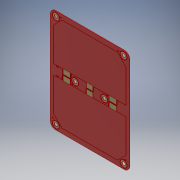
# Autodesk Inventor part: SolarPanel_PCB
Saved by Autodesk Inventor 2018 (Build 220112000, 112)
## iProperties
Created: 2018-05-13
Part Number: SolarPanel_PCB
Material: Fiberglass Batt
Document SubType Name: Modeling
Designer: Bradley
Density: 0.032 g/cm^3
Appearance: Smooth - Red
Author: Bradley
Autodesk Inventor part; units mm, degrees
ref_plane "YZ Plane" through (0, 0, 0) normal (1, 0, 0) x (0, 1, 0)
ref_plane "XZ Plane" through (0, 0, 0) normal (0, 1, 0) x (-1, 0, 0)
ref_plane "XY Plane" through (0, 0, 0) normal (0, 0, 1) x (1, 0, 0)
sketch "Sketch1" plane through (0, 0, 0) normal (0, 1, 0) x (-1, 0, 0)
  line L0 (50, 57) -> (41.5, 57) construction
  line L1 (41.5, 57) -> (41.5, -56.5) construction
  line L2 (41.5, -56.5) -> (50, -56.5) construction
  line L3 (50, -56.5) -> (50, 57) construction
  line L4 (-41.5, 57) -> (-50, 57) construction
  line L5 (-50, 57) -> (-50, -56.5) construction
  line L6 (-50, -56.5) -> (-41.5, -56.5) construction
  line L7 (-41.5, -56.5) -> (-41.5, 57) construction
  line L8 (41.5, 50) -> (-41.5, 50) construction
  line L9 (-41.5, 50) -> (-41.5, -50) construction
  line L10 (-41.5, -50) -> (41.5, -50) construction
  line L11 (41.5, -50) -> (41.5, 50) construction
  line L12 (0, 50) -> (0, -50) construction
  line L13 (33, 49.5) -> (-33, 49.5)
  line L14 (-38, 44.5) -> (-38, -44.5)
  line L15 (-33, -49.5) -> (33, -49.5)
  line L16 (38, -44.5) -> (38, 44.5)
  line L17 (34.5, 5) -> (-34.5, 5) construction
  line L18 (-34.5, 5) -> (-34.5, 36.7) construction
  line L19 (-34.5, 36.7) -> (-26.5, 44.7) construction
  line L20 (-26.5, 44.7) -> (26.5, 44.7) construction
  line L21 (26.5, 44.7) -> (34.5, 36.7) construction
  line L22 (34.5, 36.7) -> (34.5, 5) construction
  line L23 (34.5, -5) -> (-34.5, -5) construction
  line L24 (-34.5, -5) -> (-34.5, -36.7) construction
  line L25 (-34.5, -36.7) -> (-26.5, -44.7) construction
  line L26 (-26.5, -44.7) -> (26.5, -44.7) construction
  line L27 (26.5, -44.7) -> (34.5, -36.7) construction
  line L28 (34.5, -36.7) -> (34.5, -5) construction
  line L29 (0, 5) -> (0, -5) construction
  circle A0 centre (32.5, 45) radius 2.85 construction
  circle A1 centre (32.5, 45) radius 1.65
  circle A2 centre (32.5, 45) radius 1.5 construction
  line L30 (32.5, 45) -> (-32.5, 45) construction
  line L31 (-32.5, 45) -> (-32.5, -45) construction
  line L32 (-32.5, -45) -> (32.5, -45) construction
  line L33 (32.5, -45) -> (32.5, 45) construction
  circle A3 centre (-32.5, -45) radius 1.65
  circle A4 centre (32.5, -45) radius 1.65
  circle A5 centre (-32.5, 45) radius 1.65
  line L34 (14, 0) -> (-14, 0) construction
  circle A6 centre (14, 0) radius 1.65
  circle A7 centre (-14, 0) radius 1.65
  arc A8 (38, 44.5) -> (33, 49.5) centre (33, 44.5) ccw
  arc A9 (-33, 49.5) -> (-38, 44.5) centre (-33, 44.5) ccw
  arc A10 (-38, -44.5) -> (-33, -49.5) centre (-33, -44.5) ccw
  arc A11 (33, -49.5) -> (38, -44.5) centre (33, -44.5) ccw
  point P0 (0, 0)
  point P1 (0, 0)
  point P2 (38, 49.5)
  point P3 (-38, -49.5)
  point P4 (-38, 49.5)
  point P5 (38, -49.5)
  point P6 (0, 49.5)
  point P7 (0, 44.7)
  point P8 (38, 0)
  point P9 (0, 45)
  point P10 (32.5, 0)
  dimension "d0" = 100
  dimension "d1" = 8.5
  dimension "d2" = 100
  dimension "d3" = 6.5
  dimension "d4" = 7
  dimension "d5" = 12
  dimension "d6" = 10
  dimension "d7" = 69
  dimension "d8" = 39.7
  dimension "d10" = 8
  dimension "d11" = 3
  dimension "d12" = 3.3
  dimension "d13" = 5.7
  dimension "d14" = 28
  dimension "d17" = 99
  dimension "d18" = 76
  dimension "d19" = 65
  dimension "d20" = 90
  dimension "d21" = 1.6048
  dimension "d22" = 5
  constraints: 70 end point, 16 point on line, 15 parallel, 12 centre point, 12 midpoint, 9 perpendicular, 8 coincident, 8 equal radius, 8 point on circle, 8 tangent, 7 horizontal, 6 equal length, 3 vertical alignment, 2 horizontal alignment
  measures "d0" distance between parallel lines of L5 L3
  measures "d1" distance of L0.start L0.end
  measures "d2" distance between parallel lines of L10 L8
  measures "d3" distance between parallel lines of L2 L10
  measures "d4" distance between parallel lines of L8 L0
  measures "d5" distance between parallel lines of L16 L3
  measures "d6" distance between parallel lines of L23 L17
  measures "d7" distance of L17.start L17.end
  measures "d8" distance between parallel lines of L17 L20
  measures "d10" horizontal distance of L18.end L19.end
  measures "d11" diameter of A2
  measures "d12" diameter of A1
  measures "d13" diameter of A0
  measures "d14" distance of L34.start L34.end
  measures "d17" distance of point (38, -49.5) point (38, 49.5)
  measures "d18" distance of point (38, 49.5) point (-38, 49.5)
  measures "d19" distance of L30.start L30.end
  measures "d20" distance of L32.end L30.start
  measures "d21" distance edge to line of A0 L21
  measures "d22" radius of A8
extrude "Extrusion1" add sketch "Sketch1" along normal mid plane 0.5
sketch "Sketch2" plane through (0, -0.25, 0) normal (0, -1, 0) x (1, 0, 0)
  line L0 (-18.675, 5) -> (-25.675, 5)
  line L1 (-25.675, 5) -> (-25.675, 0.5)
  line L2 (-25.675, 0.5) -> (-18.675, 0.5)
  line L3 (-18.675, 0.5) -> (-18.675, 5)
  line L4 (3, 5) -> (-3, 5)
  line L5 (-3, 5) -> (-3, 0.5)
  line L6 (-3, 0.5) -> (3, 0.5)
  line L7 (3, 0.5) -> (3, 5)
  line L8 (18.675, 5) -> (25.675, 5)
  line L9 (25.675, 5) -> (25.675, 0.5)
  line L10 (25.675, 0.5) -> (18.675, 0.5)
  line L11 (18.675, 0.5) -> (18.675, 5)
  line L12 (-22.175, 5) -> (22.175, 5) construction
  line L13 (-25.675, 0) -> (25.675, 0)
  line L14 (-18.675, -5) -> (-25.675, -5)
  line L15 (-25.675, -5) -> (-25.675, -0.5)
  line L16 (-25.675, -0.5) -> (-18.675, -0.5)
  line L17 (-18.675, -0.5) -> (-18.675, -5)
  line L18 (3, -5) -> (-3, -5)
  line L19 (-3, -5) -> (-3, -0.5)
  line L20 (-3, -0.5) -> (3, -0.5)
  line L21 (3, -0.5) -> (3, -5)
  line L22 (18.675, -5) -> (25.675, -5)
  line L23 (25.675, -5) -> (25.675, -0.5)
  line L24 (25.675, -0.5) -> (18.675, -0.5)
  line L25 (18.675, -0.5) -> (18.675, -5)
  circle A0 centre (14, 0) radius 1.65 projected
  circle A1 centre (-14, 0) radius 1.65 projected
  circle A2 centre (32.5, 45) radius 1.65 projected
  circle A3 centre (-32.5, -45) radius 1.65 projected
  circle A4 centre (32.5, -45) radius 1.65 projected
  circle A5 centre (-32.5, 45) radius 1.65 projected
  line L26 (33, 49.5) -> (-33, 49.5) projected
  arc A6 (-33, 49.5) -> (-38, 44.5) centre (-33, 44.5) ccw projected
  line L27 (-38, 44.5) -> (-38, -44.5) projected
  arc A7 (-38, -44.5) -> (-33, -49.5) centre (-33, -44.5) ccw projected
  line L28 (-33, -49.5) -> (33, -49.5) projected
  arc A8 (33, -49.5) -> (38, -44.5) centre (33, -44.5) ccw projected
  line L29 (38, -44.5) -> (38, 44.5) projected
  arc A9 (38, 44.5) -> (33, 49.5) centre (33, 44.5) ccw projected
  circle A10 centre (-14, 0) radius 3
  circle A11 centre (14, 0) radius 3
  circle A12 centre (-32.5, 45) radius 3
  circle A13 centre (32.5, 45) radius 1.65 projected
  circle A14 centre (32.5, 45) radius 3
  circle A15 centre (-32.5, -45) radius 1.65 projected
  circle A16 centre (-32.5, -45) radius 3
  circle A17 centre (32.5, -45) radius 1.65 projected
  circle A18 centre (32.5, -45) radius 3
  point P0 (0, 0)
  point P1 (0, 5)
  point P2 (0, 0)
  dimension "d23" = 44.35
  dimension "d24" = 7
  dimension "d25" = 4.5
  dimension "d26" = 6
  dimension "d27" = 5
  dimension "d47" = 6
  constraints: 52 end point, 12 symmetric about line, 9 point on line, 7 coincident, 7 parallel, 6 centre point, 5 equal radius, 5 midpoint, 3 horizontal, 3 perpendicular, 2 collinear, 1 horizontal alignment, 1 vertical alignment
  measures "d23" distance of L12.end L12.start
  measures "d24" distance of L1.end L2.end
  measures "d25" distance of L0.end L1.end
  measures "d26" distance of L5.end L6.end
  measures "d27" distance from line of point (0, 0) L12
  measures "d47" diameter of A10
extrude "Extrusion2" add sketch "Sketch2" along normal blind 0.035 contours L3 L2 L1 L0 | L7 L6 L5 L4 | L8 L9 L10 L11 | A1 L13 A10 | L13 A10 A1 | A0 L13 A11 | L13 A11 A0 | L14 L15 L16 L17 | L18 L19 L20 L21 | L25 L24 L23 L22 | A12 | A14 | A16 | A18
sketch "Sketch3" plane through (0, -0.25, 0) normal (0, -1, 0) x (1, 0, 0)
  line L0 (-25.675, -5) -> (-25.675, -0.5) projected
  line L1 (-25.675, -0.5) -> (-18.675, -0.5) projected
  line L2 (-18.675, -0.5) -> (-18.675, -5) projected
  line L3 (-18.675, -5) -> (-25.675, -5) projected
  line L4 (-18.675, 5) -> (-18.675, 0.5) projected
  line L5 (-18.675, 0.5) -> (-25.675, 0.5) projected
  line L6 (-25.675, 0.5) -> (-25.675, 5) projected
  line L7 (-25.675, 5) -> (-18.675, 5) projected
  line L8 (3, 5) -> (3, 0.5) projected
  line L9 (3, 0.5) -> (-3, 0.5) projected
  line L10 (-3, 0.5) -> (-3, 5) projected
  line L11 (-3, 5) -> (3, 5) projected
  line L12 (-3, -5) -> (-3, -0.5) projected
  line L13 (-3, -0.5) -> (3, -0.5) projected
  line L14 (3, -0.5) -> (3, -5) projected
  line L15 (3, -5) -> (-3, -5) projected
  line L16 (25.675, 5) -> (25.675, 0.5) projected
  line L17 (25.675, 0.5) -> (18.675, 0.5) projected
  line L18 (18.675, 0.5) -> (18.675, 5) projected
  line L19 (18.675, 5) -> (25.675, 5) projected
  line L20 (25.675, -0.5) -> (25.675, -5) projected
  line L21 (25.675, -5) -> (18.675, -5) projected
  line L22 (18.675, -5) -> (18.675, -0.5) projected
  line L23 (18.675, -0.5) -> (25.675, -0.5) projected
  line L24 (33, 49.5) -> (-33, 49.5) projected
  arc A0 (-33, 49.5) -> (-38, 44.5) centre (-33, 44.5) ccw projected
  line L25 (-38, 44.5) -> (-38, -44.5) projected
  arc A1 (-38, -44.5) -> (-33, -49.5) centre (-33, -44.5) ccw projected
  line L26 (-33, -49.5) -> (33, -49.5) projected
  arc A2 (33, -49.5) -> (38, -44.5) centre (33, -44.5) ccw projected
  line L27 (38, -44.5) -> (38, 44.5) projected
  arc A3 (38, 44.5) -> (33, 49.5) centre (33, 44.5) ccw projected
  circle A4 centre (-18.1, 3.824) radius 0.225
  circle A5 centre (-18.1, 1.676) radius 0.225
  circle A6 centre (-18.1, 2.75) radius 0.225
  line L28 (-18.675, 5) -> (-17.7995, 4.1245)
  arc A7 (-17.675, 3.824) -> (-17.7995, 4.1245) centre (-18.1, 3.824) ccw
  line L29 (-17.675, 3.824) -> (-17.675, 1.676)
  arc A8 (-17.7995, 1.3755) -> (-17.675, 1.676) centre (-18.1, 1.676) ccw
  line L30 (-17.7995, 1.3755) -> (-18.675, 0.5)
  line L31 (-18.1, 3.824) -> (-18.1, 1.676) construction
  line L32 (-18.675, 5) -> (-18.675, 0.5)
  line L33 (3, 5) -> (3, 0.5) construction
  line L34 (3, 5) -> (3.8755, 4.1245)
  arc A9 (4, 3.824) -> (3.8755, 4.1245) centre (3.575, 3.824) ccw
  line L35 (4, 3.824) -> (4, 1.676)
  arc A10 (3.8755, 1.3755) -> (4, 1.676) centre (3.575, 1.676) ccw
  line L36 (3.8755, 1.3755) -> (3, 0.5)
  line L37 (25.675, 0.5) -> (26.5505, 1.3755)
  arc A11 (26.5505, 1.3755) -> (26.675, 1.676) centre (26.25, 1.676) ccw
  line L38 (26.675, 1.676) -> (26.675, 3.824)
  arc A12 (26.675, 3.824) -> (26.5505, 4.1245) centre (26.25, 3.824) ccw
  line L39 (26.5505, 4.1245) -> (25.675, 5)
  line L40 (3, 5) -> (3, 0.5)
  line L41 (25.675, 5) -> (25.675, 0.5)
  line L42 (-4, -3.824) -> (-4, -1.676)
  arc A13 (-4, -3.824) -> (-3.8755, -4.1245) centre (-3.575, -3.824) ccw
  arc A14 (-3.8755, -1.3755) -> (-4, -1.676) centre (-3.575, -1.676) ccw
  line L43 (-25.675, -5) -> (-25.675, -0.5)
  line L44 (-25.675, -0.5) -> (-26.5505, -1.3755)
  arc A15 (-26.675, -3.824) -> (-26.5505, -4.1245) centre (-26.25, -3.824) ccw
  line L45 (-26.675, -1.676) -> (-26.675, -3.824)
  arc A16 (-26.5505, -1.3755) -> (-26.675, -1.676) centre (-26.25, -1.676) ccw
  line L46 (-26.5505, -4.1245) -> (-25.675, -5)
  circle A17 centre (18.1, -3.824) radius 0.225
  circle A18 centre (18.1, -1.676) radius 0.225
  circle A19 centre (18.1, -2.75) radius 0.225
  line L47 (18.675, -5) -> (17.7995, -4.1245)
  arc A20 (17.675, -3.824) -> (17.7995, -4.1245) centre (18.1, -3.824) ccw
  line L48 (-3, -5) -> (-3.8755, -4.1245)
  line L49 (-3.8755, -1.3755) -> (-3, -0.5)
  line L50 (17.675, -3.824) -> (17.675, -1.676)
  arc A21 (17.7995, -1.3755) -> (17.675, -1.676) centre (18.1, -1.676) ccw
  line L51 (18.1, -3.824) -> (18.1, -1.676) construction
  line L52 (17.7995, -1.3755) -> (18.675, -0.5)
  line L53 (18.675, -5) -> (18.675, -0.5)
  line L54 (-3, -5) -> (-3, -0.5)
  line L55 (3.575, 3.824) -> (3.575, 1.676) construction
  line L56 (26.25, 3.824) -> (26.25, 1.676) construction
  line L57 (-3.575, -1.676) -> (-3.575, -3.824) construction
  line L58 (-26.25, -1.676) -> (-26.25, -3.824) construction
  circle A22 centre (3.575, 3.824) radius 0.225
  circle A23 centre (3.575, 2.75) radius 0.225
  circle A24 centre (3.575, 1.676) radius 0.225
  circle A25 centre (26.25, 3.824) radius 0.225
  circle A26 centre (26.25, 2.75) radius 0.225
  circle A27 centre (26.25, 1.676) radius 0.225
  circle A28 centre (-3.575, -1.676) radius 0.225
  circle A29 centre (-3.575, -2.75) radius 0.225
  circle A30 centre (-3.575, -3.824) radius 0.225
  circle A31 centre (-26.25, -1.676) radius 0.225
  circle A32 centre (-26.25, -2.75) radius 0.225
  circle A33 centre (-26.25, -3.824) radius 0.225
  circle A34 centre (-14, 0) radius 3 projected
  circle A35 centre (-14, 0) radius 3.5 construction
  point P0 (0, 0)
  dimension "d30" = 0.45
  dimension "d31" = 45
  dimension "d32" = 0.2
  dimension "d33" = 1
  dimension "d36" = 360
  dimension "d48" = 7
  constraints: 60 end point, 31 centre point, 24 point on circle, 19 equal radius, 15 coincident, 12 tangent, 7 equal length, 7 vertical, 5 midpoint, 2 collinear, 2 parallel, 101 other
  measures "d30" diameter of A4
  measures "d31" angle of L4 L28
  measures "d32" radial gap between concentric circles of A4 A7
  measures "d33" distance between parallel lines of L4 L29
  measures "d48" diameter of A35
extrude "Extrusion3" add sketch "Sketch3" along normal blind 0.05 contours L46 A15 L45 A16 L44 L0 | L28 A7 L29 A8 L30 L4 | L34 A9 L35 A10 L36 L8 | L48 A13 L42 A14 L49 L12 | L39 A12 L38 A11 L37 L16 | L22 L47 A20 L50 A21 L52
sketch "Sketch6" plane through (0, -0.25, 0) normal (0, -1, 0) x (1, 0, 0)
  line L0 (33, 49.5) -> (-33, 49.5) projected
  arc A0 (-33, 49.5) -> (-38, 44.5) centre (-33, 44.5) ccw projected
  line L1 (-38, 44.5) -> (-38, -44.5) projected
  arc A1 (-38, -44.5) -> (-33, -49.5) centre (-33, -44.5) ccw projected
  line L2 (-33, -49.5) -> (33, -49.5) projected
  arc A2 (33, -49.5) -> (38, -44.5) centre (33, -44.5) ccw projected
  line L3 (38, -44.5) -> (38, 44.5) projected
  arc A3 (38, 44.5) -> (33, 49.5) centre (33, 44.5) ccw projected
  line L4 (25.675, 5) -> (26.5505, 4.1245) projected
  arc A4 (26.675, 3.824) -> (26.5505, 4.1245) centre (26.25, 3.824) ccw projected
  line L5 (26.675, 3.824) -> (26.675, 1.676) projected
  arc A5 (26.5505, 1.3755) -> (26.675, 1.676) centre (26.25, 1.676) ccw projected
  line L6 (26.5505, 1.3755) -> (25.675, 0.5) projected
  line L7 (25.675, 0.5) -> (18.675, 0.5) projected
  line L8 (18.675, 0.5) -> (18.675, 5) projected
  line L9 (18.675, 5) -> (25.675, 5) projected
  circle A6 centre (32.5, -45) radius 3 projected
  circle A7 centre (32.5, 45) radius 3 projected
  circle A8 centre (14, 0) radius 3 projected
  line L10 (3, 5) -> (3.8755, 4.1245) projected
  arc A9 (4, 3.824) -> (3.8755, 4.1245) centre (3.575, 3.824) ccw projected
  line L11 (4, 3.824) -> (4, 1.676) projected
  arc A10 (3.8755, 1.3755) -> (4, 1.676) centre (3.575, 1.676) ccw projected
  line L12 (3.8755, 1.3755) -> (3, 0.5) projected
  line L13 (3, 0.5) -> (-3, 0.5) projected
  line L14 (-3, 0.5) -> (-3, 5) projected
  line L15 (-3, 5) -> (3, 5) projected
  circle A11 centre (-14, 0) radius 3 projected
  circle A12 centre (-32.5, 45) radius 3 projected
  circle A13 centre (-32.5, -45) radius 3 projected
  line L16 (-18.675, 5) -> (-17.7995, 4.1245) projected
  arc A14 (-17.675, 3.824) -> (-17.7995, 4.1245) centre (-18.1, 3.824) ccw projected
  line L17 (-17.675, 3.824) -> (-17.675, 1.676) projected
  arc A15 (-17.7995, 1.3755) -> (-17.675, 1.676) centre (-18.1, 1.676) ccw projected
  line L18 (-17.7995, 1.3755) -> (-18.675, 0.5) projected
  line L19 (-18.675, 0.5) -> (-25.675, 0.5) projected
  line L20 (-25.675, 0.5) -> (-25.675, 5) projected
  line L21 (-25.675, 5) -> (-18.675, 5) projected
  line L22 (17.7995, -1.3755) -> (18.675, -0.5) projected
  line L23 (18.675, -0.5) -> (25.675, -0.5) projected
  line L24 (25.675, -0.5) -> (25.675, -5) projected
  line L25 (25.675, -5) -> (18.675, -5) projected
  line L26 (18.675, -5) -> (17.7995, -4.1245) projected
  arc A16 (17.675, -3.824) -> (17.7995, -4.1245) centre (18.1, -3.824) ccw projected
  line L27 (17.675, -3.824) -> (17.675, -1.676) projected
  arc A17 (17.7995, -1.3755) -> (17.675, -1.676) centre (18.1, -1.676) ccw projected
  line L28 (-3.8755, -1.3755) -> (-3, -0.5) projected
  line L29 (-3, -0.5) -> (3, -0.5) projected
  line L30 (3, -0.5) -> (3, -5) projected
  line L31 (3, -5) -> (-3, -5) projected
  line L32 (-3, -5) -> (-3.8755, -4.1245) projected
  arc A18 (-4, -3.824) -> (-3.8755, -4.1245) centre (-3.575, -3.824) ccw projected
  line L33 (-4, -3.824) -> (-4, -1.676) projected
  arc A19 (-3.8755, -1.3755) -> (-4, -1.676) centre (-3.575, -1.676) ccw projected
  line L34 (-26.5505, -1.3755) -> (-25.675, -0.5) projected
  line L35 (-25.675, -0.5) -> (-18.675, -0.5) projected
  line L36 (-18.675, -0.5) -> (-18.675, -5) projected
  line L37 (-18.675, -5) -> (-25.675, -5) projected
  line L38 (-25.675, -5) -> (-26.5505, -4.1245) projected
  arc A20 (-26.675, -3.824) -> (-26.5505, -4.1245) centre (-26.25, -3.824) ccw projected
  line L39 (-26.675, -3.824) -> (-26.675, -1.676) projected
  arc A21 (-26.5505, -1.3755) -> (-26.675, -1.676) centre (-26.25, -1.676) ccw projected
  circle A22 centre (-14, 0) radius 3.5 construction
  circle A23 centre (14, 0) radius 3.5 construction
  circle A24 centre (32.5, 45) radius 1.65 construction
  circle A25 centre (32.5, 45) radius 3.5 construction
  circle A26 centre (-32.5, 45) radius 3.5 construction
  circle A27 centre (-32.5, -45) radius 1.65 construction
  circle A28 centre (-32.5, -45) radius 3.5 construction
  circle A29 centre (32.5, -45) radius 1.65 construction
  circle A30 centre (32.5, -45) radius 3.5 construction
  line L40 (-34.75, 4.75) -> (-25.925, 4.75) construction
  line L41 (-25.925, 4.75) -> (-25.925, 0.25) construction
  line L42 (-25.925, 0.25) -> (-18.425, 0.25) construction
  line L43 (-18.425, 0.25) -> (-18.425, 4.75) construction
  line L44 (-18.425, 4.75) -> (-3.25, 4.75) construction
  line L45 (-3.25, 4.75) -> (-3.25, 0.25) construction
  line L46 (-3.25, 0.25) -> (3.25, 0.25) construction
  line L47 (3.25, 0.25) -> (3.25, 4.75) construction
  line L48 (3.25, 4.75) -> (18.425, 4.75) construction
  line L49 (18.425, 4.75) -> (18.425, 0.25) construction
  line L50 (18.425, 0.25) -> (25.925, 0.25) construction
  line L51 (25.925, 0.25) -> (25.925, 4.75) construction
  line L52 (25.925, 4.75) -> (34.75, 4.75) construction
  line L53 (34.75, 4.75) -> (34.75, 36.8036) construction
  line L54 (34.75, 36.8036) -> (26.6036, 44.95) construction
  line L55 (26.6036, 44.95) -> (-26.6036, 44.95) construction
  line L56 (-26.6036, 44.95) -> (-34.75, 36.8036) construction
  line L57 (-34.75, 36.8036) -> (-34.75, 4.75) construction
  line L58 (-25.675, 0.5) -> (-18.675, 0.5) construction
  line L59 (-3, 0.5) -> (3, 0.5) construction
  line L60 (18.675, 0.5) -> (25.675, 0.5) construction
  line L61 (-34.5, 36.7) -> (-34.5, 5) construction
  line L62 (-26.5, 44.7) -> (-34.5, 36.7) construction
  line L63 (26.5, 44.7) -> (-26.5, 44.7) construction
  line L64 (34.5, 36.7) -> (26.5, 44.7) construction
  line L65 (34.5, 5) -> (34.5, 36.7) construction
  line L66 (-26.6346, 45.025) -> (26.6346, 45.025)
  line L67 (26.6346, 45.025) -> (34.825, 36.8346)
  line L68 (34.825, 36.8346) -> (34.825, 4.675)
  line L69 (34.825, 4.675) -> (26, 4.675)
  line L70 (26, 4.675) -> (26, 0.175)
  line L71 (26, 0.175) -> (18.35, 0.175)
  line L72 (18.35, 0.175) -> (18.35, 4.675)
  line L73 (18.35, 4.675) -> (3.325, 4.675)
  line L74 (3.325, 4.675) -> (3.325, 0.175)
  line L75 (3.325, 0.175) -> (-3.325, 0.175)
  line L76 (-3.325, 0.175) -> (-3.325, 4.675)
  line L77 (-3.325, 4.675) -> (-18.35, 4.675)
  line L78 (-18.35, 4.675) -> (-18.35, 0.175)
  line L79 (-18.35, 0.175) -> (-26, 0.175)
  line L80 (-26, 0.175) -> (-26, 4.675)
  line L81 (-26, 4.675) -> (-34.825, 4.675)
  line L82 (-34.825, 4.675) -> (-34.825, 36.8346)
  line L83 (-34.825, 36.8346) -> (-26.6346, 45.025)
  line L84 (-26.5725, 44.875) -> (26.5725, 44.875)
  line L85 (26.5725, 44.875) -> (34.675, 36.7725)
  line L86 (34.675, 36.7725) -> (34.675, 4.825)
  line L87 (34.675, 4.825) -> (25.85, 4.825)
  line L88 (25.85, 4.825) -> (25.85, 0.325)
  line L89 (25.85, 0.325) -> (18.5, 0.325)
  line L90 (18.5, 0.325) -> (18.5, 4.825)
  line L91 (18.5, 4.825) -> (3.175, 4.825)
  line L92 (3.175, 4.825) -> (3.175, 0.325)
  line L93 (3.175, 0.325) -> (-3.175, 0.325)
  line L94 (-3.175, 0.325) -> (-3.175, 4.825)
  line L95 (-3.175, 4.825) -> (-18.5, 4.825)
  line L96 (-18.5, 4.825) -> (-18.5, 0.325)
  line L97 (-18.5, 0.325) -> (-25.85, 0.325)
  line L98 (-25.85, 0.325) -> (-25.85, 4.825)
  line L99 (-25.85, 4.825) -> (-34.675, 4.825)
  line L100 (-34.675, 4.825) -> (-34.675, 36.7725)
  line L101 (-34.675, 36.7725) -> (-26.5725, 44.875)
  line L102 (-14, 0) -> (14, 0) construction
  line L103 (-34.675, -4.825) -> (-25.85, -4.825)
  line L104 (-34.825, -4.675) -> (-26, -4.675)
  line L105 (-34.675, -36.7725) -> (-34.675, -4.825)
  line L106 (-34.825, -36.8346) -> (-34.825, -4.675)
  line L107 (-34.75, -4.75) -> (-34.75, -36.8036) construction
  line L108 (-25.925, -4.75) -> (-34.75, -4.75) construction
  line L109 (3.325, -4.675) -> (18.35, -4.675)
  line L110 (18.425, -4.75) -> (3.25, -4.75) construction
  line L111 (3.175, -4.825) -> (18.5, -4.825)
  line L112 (3.25, -4.75) -> (3.25, -0.25) construction
  line L113 (3.25, -0.25) -> (-3.25, -0.25) construction
  line L114 (-3.325, -0.175) -> (3.325, -0.175)
  line L115 (-25.85, -4.825) -> (-25.85, -0.325)
  line L116 (-25.85, -0.325) -> (-18.5, -0.325)
  line L117 (-3.325, -4.675) -> (-3.325, -0.175)
  line L118 (-18.35, -4.675) -> (-3.325, -4.675)
  line L119 (-18.35, -0.175) -> (-18.35, -4.675)
  line L120 (-18.5, -0.325) -> (-18.5, -4.825)
  line L121 (-18.5, -4.825) -> (-3.175, -4.825)
  line L122 (-3.175, -4.825) -> (-3.175, -0.325)
  line L123 (-3.25, -0.25) -> (-3.25, -4.75) construction
  line L124 (-3.25, -4.75) -> (-18.425, -4.75) construction
  line L125 (-18.425, -4.75) -> (-18.425, -0.25) construction
  line L126 (-25.925, -0.25) -> (-25.925, -4.75) construction
  line L127 (-26, -4.675) -> (-26, -0.175)
  line L128 (-18.425, -0.25) -> (-25.925, -0.25) construction
  line L129 (18.425, -0.25) -> (18.425, -4.75) construction
  line L130 (18.35, -4.675) -> (18.35, -0.175)
  line L131 (18.5, -0.325) -> (25.85, -0.325)
  line L132 (25.925, -0.25) -> (18.425, -0.25) construction
  line L133 (18.35, -0.175) -> (26, -0.175)
  line L134 (25.85, -0.325) -> (25.85, -4.825)
  line L135 (25.925, -4.75) -> (25.925, -0.25) construction
  line L136 (26, -0.175) -> (26, -4.675)
  line L137 (26.6346, -45.025) -> (-26.6346, -45.025)
  line L138 (34.675, -4.825) -> (34.675, -36.7725)
  line L139 (34.75, -36.8036) -> (34.75, -4.75) construction
  line L140 (34.825, -4.675) -> (34.825, -36.8346)
  line L141 (18.5, -4.825) -> (18.5, -0.325)
  line L142 (26.5725, -44.875) -> (-26.5725, -44.875)
  line L143 (-26.6036, -44.95) -> (26.6036, -44.95) construction
  line L144 (34.75, -4.75) -> (25.925, -4.75) construction
  line L145 (25.85, -4.825) -> (34.675, -4.825)
  line L146 (26, -4.675) -> (34.825, -4.675)
  line L147 (-26, -0.175) -> (-18.35, -0.175)
  line L148 (34.675, -36.7725) -> (26.5725, -44.875)
  line L149 (26.6036, -44.95) -> (34.75, -36.8036) construction
  line L150 (34.825, -36.8346) -> (26.6346, -45.025)
  line L151 (-26.5725, -44.875) -> (-34.675, -36.7725)
  line L152 (-34.75, -36.8036) -> (-26.6036, -44.95) construction
  line L153 (-26.6346, -45.025) -> (-34.825, -36.8346)
  line L154 (3.175, -0.325) -> (3.175, -4.825)
  line L155 (3.325, -0.175) -> (3.325, -4.675)
  line L156 (-3.175, -0.325) -> (3.175, -0.325)
  circle A31 centre (-14, 0) radius 3.575
  circle A32 centre (-14, 0) radius 3.425
  circle A33 centre (14, 0) radius 3.575
  circle A34 centre (14, 0) radius 3.425
  circle A35 centre (32.5, 45) radius 3.575
  circle A36 centre (32.5, 45) radius 3.425
  circle A37 centre (-32.5, 45) radius 3.575
  circle A38 centre (-32.5, 45) radius 3.425
  circle A39 centre (32.5, -45) radius 3.575
  circle A40 centre (32.5, -45) radius 3.425
  circle A41 centre (-32.5, -45) radius 3.575
  circle A42 centre (-32.5, -45) radius 3.425
  line L157 (-32.0298, 4.2303) -> (-29.8638, 4.2303) construction
  line L158 (-29.8638, 4.2303) -> (-29.8638, 3.4284) construction
  line L159 (-29.8638, 3.4284) -> (-32.0298, 3.4284) construction
  line L160 (-32.0298, 3.4284) -> (-32.0298, 4.2303) construction
  line L161 (-32.0692, -3.4048) -> (-29.9032, -3.4048) construction
  line L162 (-29.9032, -3.4048) -> (-29.9032, -4.2067) construction
  line L163 (-29.9032, -4.2067) -> (-32.0692, -4.2067) construction
  line L164 (-32.0692, -4.2067) -> (-32.0692, -3.4048) construction
  line L165 (-17.5305, -3.2221) -> (-15.3645, -3.2221) construction
  line L166 (-15.3645, -3.2221) -> (-15.3645, -4.024) construction
  line L167 (-15.3645, -4.024) -> (-17.5305, -4.024) construction
  line L168 (-17.5305, -4.024) -> (-17.5305, -3.2221) construction
  line L169 (15.9624, 4.2512) -> (18.1284, 4.2512) construction
  line L170 (18.1284, 4.2512) -> (18.1284, 3.4492) construction
  line L171 (18.1284, 3.4492) -> (15.9624, 3.4492) construction
  line L172 (15.9624, 3.4492) -> (15.9624, 4.2512) construction
  line L173 (-28.7606, 46.6145) -> (-26.5946, 46.6145) construction
  line L174 (-26.5946, 46.6145) -> (-26.5946, 45.8126) construction
  line L175 (-26.5946, 45.8126) -> (-28.7606, 45.8126) construction
  line L176 (-28.7606, 45.8126) -> (-28.7606, 46.6145) construction
  line L177 (26.5067, 46.7387) -> (28.6727, 46.7387) construction
  line L178 (28.6727, 46.7387) -> (28.6727, 45.9367) construction
  line L179 (28.6727, 45.9367) -> (26.5067, 45.9367) construction
  line L180 (26.5067, 45.9367) -> (26.5067, 46.7387) construction
  line L181 (-36.2344, -40.3855) -> (-34.0684, -40.3855) construction
  line L182 (-34.0684, -40.3855) -> (-34.0684, -41.1874) construction
  line L183 (-34.0684, -41.1874) -> (-36.2344, -41.1874) construction
  line L184 (-36.2344, -41.1874) -> (-36.2344, -40.3855) construction
  line L185 (33.6109, -40.4304) -> (35.7769, -40.4304) construction
  line L186 (35.7769, -40.4304) -> (35.7769, -41.2324) construction
  line L187 (35.7769, -41.2324) -> (33.6109, -41.2324) construction
  line L188 (33.6109, -41.2324) -> (33.6109, -40.4304) construction
  line L189 (-28.0027, 45.8126) -> (-28.2037, 45.8126)
  line L190 (-28.2037, 45.8126) -> (-28.2037, 46.1672)
  line L191 (-28.2037, 46.1672) -> (-28.4766, 46.1672)
  line L192 (-28.4766, 46.1672) -> (-28.4766, 45.8126)
  line L193 (-28.4766, 45.8126) -> (-28.6776, 45.8126)
  line L194 (-28.6776, 45.8126) -> (-28.6776, 46.6126)
  line L195 (-28.6776, 46.6126) -> (-28.4766, 46.6126)
  line L196 (-28.4766, 46.6126) -> (-28.4766, 46.3196)
  line L197 (-28.4766, 46.3196) -> (-28.2037, 46.3196)
  line L198 (-28.2037, 46.3196) -> (-28.2037, 46.6126)
  line L199 (-28.2037, 46.6126) -> (-28.0027, 46.6126)
  line L200 (-28.0027, 46.6126) -> (-28.0027, 45.8126)
  line L201 (-27.2863, 45.8126) -> (-27.8147, 45.8126)
  line L202 (-27.8147, 45.8126) -> (-27.8147, 45.952)
  line L203 (-27.8147, 45.952) -> (-27.6461, 45.952)
  line L204 (-27.6461, 45.952) -> (-27.6461, 46.3753)
  line L205 (-27.6461, 46.3753) -> (-27.8147, 46.3753)
  line L206 (-27.8147, 46.3753) -> (-27.8147, 46.5056)
  spline S0 degree 2 poles (-27.8147, 46.5056) (-27.7777, 46.5056) (-27.7045, 46.5154) (-27.6824, 46.5257) knots 0 0 0 1 2 2 2
  spline S1 degree 2 poles (-27.6824, 46.5257) (-27.6571, 46.5387) (-27.6286, 46.5821) (-27.626, 46.6145) knots 0 0 0 1 2 2 2
  line L207 (-27.626, 46.6145) -> (-27.451, 46.6145)
  line L208 (-27.451, 46.6145) -> (-27.451, 45.952)
  line L209 (-27.451, 45.952) -> (-27.2863, 45.952)
  line L210 (-27.2863, 45.952) -> (-27.2863, 45.8126)
  line L211 (27.2646, 45.9231) -> (27.0636, 45.9231)
  line L212 (27.0636, 45.9231) -> (27.0636, 46.2777)
  line L213 (27.0636, 46.2777) -> (26.7907, 46.2777)
  line L214 (26.7907, 46.2777) -> (26.7907, 45.9231)
  line L215 (26.7907, 45.9231) -> (26.5897, 45.9231)
  line L216 (26.5897, 45.9231) -> (26.5897, 46.7231)
  line L217 (26.5897, 46.7231) -> (26.7907, 46.7231)
  line L218 (26.7907, 46.7231) -> (26.7907, 46.4301)
  line L219 (26.7907, 46.4301) -> (27.0636, 46.4301)
  line L220 (27.0636, 46.4301) -> (27.0636, 46.7231)
  line L221 (27.0636, 46.7231) -> (27.2646, 46.7231)
  line L222 (27.2646, 46.7231) -> (27.2646, 45.9231)
  line L223 (28.0166, 45.9231) -> (27.4286, 45.9231)
  line L224 (27.4286, 45.9231) -> (27.4286, 46.0534)
  spline S2 degree 2 poles (27.4286, 46.0534) (27.5032, 46.1131) (27.6224, 46.2181) (27.6672, 46.2654) knots 0 0 0 1 2 2 2
  spline S3 degree 2 poles (27.6672, 46.2654) (27.7262, 46.327) (27.7787, 46.421) (27.7787, 46.4703) knots 0 0 0 1 2 2 2
  spline S4 degree 2 poles (27.7787, 46.4703) (27.7787, 46.526) (27.7119, 46.5857) (27.6523, 46.5857) knots 0 0 0 1 2 2 2
  spline S5 degree 2 poles (27.6523, 46.5857) (27.6218, 46.5857) (27.5673, 46.5708) (27.5395, 46.5591) knots 0 0 0 1 2 2 2
  spline S6 degree 2 poles (27.5395, 46.5591) (27.5122, 46.5468) (27.4733, 46.5209) (27.4636, 46.5144) knots 0 0 0 1 2 2 2
  line L225 (27.4636, 46.5144) -> (27.448, 46.5144)
  line L226 (27.448, 46.5144) -> (27.448, 46.6888)
  spline S7 degree 2 poles (27.448, 46.6888) (27.4818, 46.705) (27.6257, 46.7387) (27.6925, 46.7387) knots 0 0 0 1 2 2 2
  spline S8 degree 2 poles (27.6925, 46.7387) (27.8351, 46.7387) (27.9816, 46.6116) (27.9816, 46.4969) knots 0 0 0 1 2 2 2
  spline S9 degree 2 poles (27.9816, 46.4969) (27.9816, 46.4262) (27.9148, 46.2901) (27.8377, 46.2123) knots 0 0 0 1 2 2 2
  spline S10 degree 2 poles (27.8377, 46.2123) (27.7891, 46.1643) (27.6976, 46.0897) (27.6775, 46.0742) knots 0 0 0 1 2 2 2
  line L227 (27.6775, 46.0742) -> (28.0166, 46.0742)
  line L228 (28.0166, 46.0742) -> (28.0166, 45.9231)
  line L229 (16.7203, 3.4512) -> (16.5193, 3.4512)
  line L230 (16.5193, 3.4512) -> (16.5193, 3.8058)
  line L231 (16.5193, 3.8058) -> (16.2464, 3.8058)
  line L232 (16.2464, 3.8058) -> (16.2464, 3.4512)
  line L233 (16.2464, 3.4512) -> (16.0454, 3.4512)
  line L234 (16.0454, 3.4512) -> (16.0454, 4.2512)
  line L235 (16.0454, 4.2512) -> (16.2464, 4.2512)
  line L236 (16.2464, 4.2512) -> (16.2464, 3.9581)
  line L237 (16.2464, 3.9581) -> (16.5193, 3.9581)
  line L238 (16.5193, 3.9581) -> (16.5193, 4.2512)
  line L239 (16.5193, 4.2512) -> (16.7203, 4.2512)
  line L240 (16.7203, 4.2512) -> (16.7203, 3.4512)
  line L241 (17.482, 3.6379) -> (17.3738, 3.6379)
  line L242 (17.3738, 3.6379) -> (17.3738, 3.4492)
  line L243 (17.3738, 3.4492) -> (17.1799, 3.4492)
  line L244 (17.1799, 3.4492) -> (17.1799, 3.6379)
  line L245 (17.1799, 3.6379) -> (16.8273, 3.6379)
  line L246 (16.8273, 3.6379) -> (16.8273, 3.787)
  line L247 (16.8273, 3.787) -> (17.1734, 4.2512)
  line L248 (17.1734, 4.2512) -> (17.3738, 4.2512)
  line L249 (17.3738, 4.2512) -> (17.3738, 3.7818)
  line L250 (17.3738, 3.7818) -> (17.482, 3.7818)
  line L251 (17.482, 3.7818) -> (17.482, 3.6379)
  line L252 (17.1799, 3.7818) -> (17.1799, 4.0541)
  line L253 (17.1799, 4.0541) -> (16.977, 3.7818)
  line L254 (16.977, 3.7818) -> (17.1799, 3.7818)
  line L255 (-16.7726, -4.0389) -> (-16.9736, -4.0389)
  line L256 (-16.9736, -4.0389) -> (-16.9736, -3.6843)
  line L257 (-16.9736, -3.6843) -> (-17.2465, -3.6843)
  line L258 (-17.2465, -3.6843) -> (-17.2465, -4.0389)
  line L259 (-17.2465, -4.0389) -> (-17.4475, -4.0389)
  line L260 (-17.4475, -4.0389) -> (-17.4475, -3.2389)
  line L261 (-17.4475, -3.2389) -> (-17.2465, -3.2389)
  line L262 (-17.2465, -3.2389) -> (-17.2465, -3.532)
  line L263 (-17.2465, -3.532) -> (-16.9736, -3.532)
  line L264 (-16.9736, -3.532) -> (-16.9736, -3.2389)
  line L265 (-16.9736, -3.2389) -> (-16.7726, -3.2389)
  line L266 (-16.7726, -3.2389) -> (-16.7726, -4.0389)
  spline S11 degree 2 poles (-16.0407, -3.7965) (-16.0407, -3.8555) (-16.0841, -3.9521) (-16.1263, -3.9858) knots 0 0 0 1 2 2 2
  spline S12 degree 2 poles (-16.1263, -3.9858) (-16.1684, -4.0195) (-16.2831, -4.0558) (-16.3655, -4.0558) knots 0 0 0 1 2 2 2
  spline S13 degree 2 poles (-16.3655, -4.0558) (-16.4588, -4.0558) (-16.5924, -4.0247) (-16.6345, -4.0052) knots 0 0 0 1 2 2 2
  line L267 (-16.6345, -4.0052) -> (-16.6345, -3.8315)
  line L268 (-16.6345, -3.8315) -> (-16.6151, -3.8315)
  spline S14 degree 2 poles (-16.6151, -3.8315) (-16.571, -3.8594) (-16.4524, -3.9009) (-16.4031, -3.9009) knots 0 0 0 1 2 2 2
  spline S15 degree 2 poles (-16.4031, -3.9009) (-16.3739, -3.9009) (-16.3058, -3.8905) (-16.2825, -3.8736) knots 0 0 0 1 2 2 2
  spline S16 degree 2 poles (-16.2825, -3.8736) (-16.2643, -3.86) (-16.2423, -3.8205) (-16.2423, -3.7848) knots 0 0 0 1 2 2 2
  spline S17 degree 2 poles (-16.2423, -3.7848) (-16.2423, -3.7491) (-16.2734, -3.7109) (-16.2994, -3.7018) knots 0 0 0 1 2 2 2
  spline S18 degree 2 poles (-16.2994, -3.7018) (-16.3253, -3.6927) (-16.3972, -3.6908) (-16.4251, -3.6908) knots 0 0 0 1 2 2 2
  line L269 (-16.4251, -3.6908) -> (-16.4595, -3.6908)
  line L270 (-16.4595, -3.6908) -> (-16.4595, -3.5501)
  line L271 (-16.4595, -3.5501) -> (-16.4277, -3.5501)
  spline S19 degree 2 poles (-16.4277, -3.5501) (-16.3914, -3.5501) (-16.3298, -3.5436) (-16.3084, -3.5339) knots 0 0 0 1 2 2 2
  spline S20 degree 2 poles (-16.3084, -3.5339) (-16.287, -3.5235) (-16.263, -3.4872) (-16.263, -3.4561) knots 0 0 0 1 2 2 2
  spline S21 degree 2 poles (-16.263, -3.4561) (-16.263, -3.4315) (-16.2857, -3.401) (-16.3019, -3.3926) knots 0 0 0 1 2 2 2
  spline S22 degree 2 poles (-16.3019, -3.3926) (-16.3214, -3.3829) (-16.3733, -3.3764) (-16.3914, -3.3764) knots 0 0 0 1 2 2 2
  spline S23 degree 2 poles (-16.3914, -3.3764) (-16.4206, -3.3764) (-16.4822, -3.39) (-16.5107, -3.401) knots 0 0 0 1 2 2 2
  spline S24 degree 2 poles (-16.5107, -3.401) (-16.5334, -3.4094) (-16.5827, -3.4367) (-16.5943, -3.4438) knots 0 0 0 1 2 2 2
  line L272 (-16.5943, -3.4438) -> (-16.6112, -3.4438)
  line L273 (-16.6112, -3.4438) -> (-16.6112, -3.2726)
  spline S25 degree 2 poles (-16.6112, -3.2726) (-16.5697, -3.2551) (-16.4297, -3.2221) (-16.3564, -3.2221) knots 0 0 0 1 2 2 2
  spline S26 degree 2 poles (-16.3564, -3.2221) (-16.2851, -3.2221) (-16.1801, -3.2467) (-16.1431, -3.2707) knots 0 0 0 1 2 2 2
  spline S27 degree 2 poles (-16.1431, -3.2707) (-16.1023, -3.296) (-16.0614, -3.3738) (-16.0614, -3.4224) knots 0 0 0 1 2 2 2
  spline S28 degree 2 poles (-16.0614, -3.4224) (-16.0614, -3.4911) (-16.1405, -3.5936) (-16.2053, -3.6085) knots 0 0 0 1 2 2 2
  line L274 (-16.2053, -3.6085) -> (-16.2053, -3.6162)
  spline S29 degree 2 poles (-16.2053, -3.6162) (-16.1768, -3.6201) (-16.1224, -3.6409) (-16.0964, -3.6642) knots 0 0 0 1 2 2 2
  spline S30 degree 2 poles (-16.0964, -3.6642) (-16.0724, -3.685) (-16.0407, -3.7511) (-16.0407, -3.7965) knots 0 0 0 1 2 2 2
  spline S31 degree 2 poles (-31.371, -3.6725) (-31.371, -3.7283) (-31.4066, -3.8294) (-31.4397, -3.8631) knots 0 0 0 1 2 2 2
  spline S32 degree 2 poles (-31.4397, -3.8631) (-31.4598, -3.8845) (-31.5091, -3.9195) (-31.5382, -3.9318) knots 0 0 0 1 2 2 2
  spline S33 degree 2 poles (-31.5382, -3.9318) (-31.5681, -3.9441) (-31.6374, -3.9584) (-31.6802, -3.9584) knots 0 0 0 1 2 2 2
  line L275 (-31.6802, -3.9584) -> (-31.7852, -3.9584)
  line L276 (-31.7852, -3.9584) -> (-31.7852, -4.2203)
  line L277 (-31.7852, -4.2203) -> (-31.9862, -4.2203)
  line L278 (-31.9862, -4.2203) -> (-31.9862, -3.4203)
  line L279 (-31.9862, -3.4203) -> (-31.6757, -3.4203)
  spline S34 degree 2 poles (-31.6757, -3.4203) (-31.607, -3.4203) (-31.5065, -3.4456) (-31.4656, -3.4728) knots 0 0 0 1 2 2 2
  spline S35 degree 2 poles (-31.4656, -3.4728) (-31.4202, -3.5033) (-31.371, -3.6031) (-31.371, -3.6725) knots 0 0 0 1 2 2 2
  spline S36 degree 2 poles (-31.5771, -3.6777) (-31.5771, -3.6433) (-31.6096, -3.5947) (-31.6316, -3.5856) knots 0 0 0 1 2 2 2
  spline S37 degree 2 poles (-31.6316, -3.5856) (-31.6601, -3.5733) (-31.712, -3.5694) (-31.7567, -3.5694) knots 0 0 0 1 2 2 2
  line L280 (-31.7567, -3.5694) -> (-31.7852, -3.5694)
  line L281 (-31.7852, -3.5694) -> (-31.7852, -3.8093)
  line L282 (-31.7852, -3.8093) -> (-31.771, -3.8093)
  spline S38 degree 2 poles (-31.771, -3.8093) (-31.7431, -3.8093) (-31.6925, -3.808) (-31.6737, -3.8048) knots 0 0 0 1 2 2 2
  spline S39 degree 2 poles (-31.6737, -3.8048) (-31.6575, -3.8022) (-31.6219, -3.7866) (-31.6121, -3.7769) knots 0 0 0 1 2 2 2
  spline S40 degree 2 poles (-31.6121, -3.7769) (-31.5914, -3.7574) (-31.5771, -3.714) (-31.5771, -3.6777) knots 0 0 0 1 2 2 2
  line L283 (-30.5956, -3.4203) -> (-30.8705, -4.2203)
  line L284 (-30.8705, -4.2203) -> (-31.0799, -4.2203)
  line L285 (-31.0799, -4.2203) -> (-31.3548, -3.4203)
  line L286 (-31.3548, -3.4203) -> (-31.1467, -3.4203)
  line L287 (-31.1467, -3.4203) -> (-30.9723, -3.9629)
  line L288 (-30.9723, -3.9629) -> (-30.7985, -3.4203)
  line L289 (-30.7985, -3.4203) -> (-30.5956, -3.4203)
  line L290 (-29.935, -4.2203) -> (-30.523, -4.2203)
  line L291 (-30.523, -4.2203) -> (-30.523, -4.09)
  spline S41 degree 2 poles (-30.523, -4.09) (-30.4484, -4.0304) (-30.3292, -3.9253) (-30.2844, -3.878) knots 0 0 0 1 2 2 2
  spline S42 degree 2 poles (-30.2844, -3.878) (-30.2254, -3.8164) (-30.1729, -3.7224) (-30.1729, -3.6731) knots 0 0 0 1 2 2 2
  spline S43 degree 2 poles (-30.1729, -3.6731) (-30.1729, -3.6174) (-30.2397, -3.5577) (-30.2993, -3.5577) knots 0 0 0 1 2 2 2
  spline S44 degree 2 poles (-30.2993, -3.5577) (-30.3298, -3.5577) (-30.3843, -3.5727) (-30.4121, -3.5843) knots 0 0 0 1 2 2 2
  spline S45 degree 2 poles (-30.4121, -3.5843) (-30.4394, -3.5966) (-30.4783, -3.6226) (-30.488, -3.6291) knots 0 0 0 1 2 2 2
  line L292 (-30.488, -3.6291) -> (-30.5036, -3.6291)
  line L293 (-30.5036, -3.6291) -> (-30.5036, -3.4547)
  spline S46 degree 2 poles (-30.5036, -3.4547) (-30.4698, -3.4385) (-30.3259, -3.4048) (-30.2591, -3.4048) knots 0 0 0 1 2 2 2
  spline S47 degree 2 poles (-30.2591, -3.4048) (-30.1165, -3.4048) (-29.97, -3.5318) (-29.97, -3.6466) knots 0 0 0 1 2 2 2
  spline S48 degree 2 poles (-29.97, -3.6466) (-29.97, -3.7172) (-30.0368, -3.8534) (-30.1139, -3.9312) knots 0 0 0 1 2 2 2
  spline S49 degree 2 poles (-30.1139, -3.9312) (-30.1625, -3.9791) (-30.254, -4.0537) (-30.2741, -4.0693) knots 0 0 0 1 2 2 2
  line L294 (-30.2741, -4.0693) -> (-29.935, -4.0693)
  line L295 (-29.935, -4.0693) -> (-29.935, -4.2203)
  spline S50 degree 2 poles (-31.3316, 3.9762) (-31.3316, 3.9205) (-31.3672, 3.8193) (-31.4003, 3.7856) knots 0 0 0 1 2 2 2
  spline S51 degree 2 poles (-31.4003, 3.7856) (-31.4204, 3.7642) (-31.4697, 3.7292) (-31.4988, 3.7169) knots 0 0 0 1 2 2 2
  spline S52 degree 2 poles (-31.4988, 3.7169) (-31.5286, 3.7046) (-31.598, 3.6903) (-31.6408, 3.6903) knots 0 0 0 1 2 2 2
  line L296 (-31.6408, 3.6903) -> (-31.7458, 3.6903)
  line L297 (-31.7458, 3.6903) -> (-31.7458, 3.4284)
  line L298 (-31.7458, 3.4284) -> (-31.9468, 3.4284)
  line L299 (-31.9468, 3.4284) -> (-31.9468, 4.2284)
  line L300 (-31.9468, 4.2284) -> (-31.6363, 4.2284)
  spline S53 degree 2 poles (-31.6363, 4.2284) (-31.5675, 4.2284) (-31.4671, 4.2031) (-31.4262, 4.1759) knots 0 0 0 1 2 2 2
  spline S54 degree 2 poles (-31.4262, 4.1759) (-31.3808, 4.1454) (-31.3316, 4.0456) (-31.3316, 3.9762) knots 0 0 0 1 2 2 2
  spline S55 degree 2 poles (-31.5377, 3.971) (-31.5377, 4.0054) (-31.5701, 4.054) (-31.5922, 4.0631) knots 0 0 0 1 2 2 2
  spline S56 degree 2 poles (-31.5922, 4.0631) (-31.6207, 4.0754) (-31.6726, 4.0793) (-31.7173, 4.0793) knots 0 0 0 1 2 2 2
  line L301 (-31.7173, 4.0793) -> (-31.7458, 4.0793)
  line L302 (-31.7458, 4.0793) -> (-31.7458, 3.8394)
  line L303 (-31.7458, 3.8394) -> (-31.7316, 3.8394)
  spline S57 degree 2 poles (-31.7316, 3.8394) (-31.7037, 3.8394) (-31.6531, 3.8407) (-31.6343, 3.844) knots 0 0 0 1 2 2 2
  spline S58 degree 2 poles (-31.6343, 3.844) (-31.6181, 3.8466) (-31.5825, 3.8621) (-31.5727, 3.8718) knots 0 0 0 1 2 2 2
  spline S59 degree 2 poles (-31.5727, 3.8718) (-31.552, 3.8913) (-31.5377, 3.9347) (-31.5377, 3.971) knots 0 0 0 1 2 2 2
  line L304 (-30.5562, 4.2284) -> (-30.8311, 3.4284)
  line L305 (-30.8311, 3.4284) -> (-31.0405, 3.4284)
  line L306 (-31.0405, 3.4284) -> (-31.3154, 4.2284)
  line L307 (-31.3154, 4.2284) -> (-31.1073, 4.2284)
  line L308 (-31.1073, 4.2284) -> (-30.9329, 3.6858)
  line L309 (-30.9329, 3.6858) -> (-30.7591, 4.2284)
  line L310 (-30.7591, 4.2284) -> (-30.5562, 4.2284)
  line L311 (-29.9312, 3.4284) -> (-30.4596, 3.4284)
  line L312 (-30.4596, 3.4284) -> (-30.4596, 3.5678)
  line L313 (-30.4596, 3.5678) -> (-30.291, 3.5678)
  line L314 (-30.291, 3.5678) -> (-30.291, 3.9911)
  line L315 (-30.291, 3.9911) -> (-30.4596, 3.9911)
  line L316 (-30.4596, 3.9911) -> (-30.4596, 4.1214)
  spline S60 degree 2 poles (-30.4596, 4.1214) (-30.4227, 4.1214) (-30.3494, 4.1312) (-30.3274, 4.1415) knots 0 0 0 1 2 2 2
  spline S61 degree 2 poles (-30.3274, 4.1415) (-30.3021, 4.1545) (-30.2735, 4.1979) (-30.271, 4.2303) knots 0 0 0 1 2 2 2
  line L317 (-30.271, 4.2303) -> (-30.0959, 4.2303)
  line L318 (-30.0959, 4.2303) -> (-30.0959, 3.5678)
  line L319 (-30.0959, 3.5678) -> (-29.9312, 3.5678)
  line L320 (-29.9312, 3.5678) -> (-29.9312, 3.4284)
  line L321 (-35.4765, -41.1855) -> (-35.6775, -41.1855)
  line L322 (-35.6775, -41.1855) -> (-35.6775, -40.8309)
  line L323 (-35.6775, -40.8309) -> (-35.9504, -40.8309)
  line L324 (-35.9504, -40.8309) -> (-35.9504, -41.1855)
  line L325 (-35.9504, -41.1855) -> (-36.1514, -41.1855)
  line L326 (-36.1514, -41.1855) -> (-36.1514, -40.3855)
  line L327 (-36.1514, -40.3855) -> (-35.9504, -40.3855)
  line L328 (-35.9504, -40.3855) -> (-35.9504, -40.6785)
  line L329 (-35.9504, -40.6785) -> (-35.6775, -40.6785)
  line L330 (-35.6775, -40.6785) -> (-35.6775, -40.3855)
  line L331 (-35.6775, -40.3855) -> (-35.4765, -40.3855)
  line L332 (-35.4765, -40.3855) -> (-35.4765, -41.1855)
  spline S62 degree 2 poles (-34.7426, -40.9145) (-34.7426, -40.9774) (-34.7854, -41.0837) (-34.8276, -41.122) knots 0 0 0 1 2 2 2
  spline S63 degree 2 poles (-34.8276, -41.122) (-34.8697, -41.1602) (-34.9851, -41.2023) (-35.0694, -41.2023) knots 0 0 0 1 2 2 2
  spline S64 degree 2 poles (-35.0694, -41.2023) (-35.1588, -41.2017) (-35.2872, -41.1725) (-35.3293, -41.1537) knots 0 0 0 1 2 2 2
  line L333 (-35.3293, -41.1537) -> (-35.3293, -40.9793)
  line L334 (-35.3293, -40.9793) -> (-35.3112, -40.9793)
  spline S65 degree 2 poles (-35.3112, -40.9793) (-35.2956, -40.9878) (-35.258, -41.0098) (-35.2276, -41.0215) knots 0 0 0 1 2 2 2
  spline S66 degree 2 poles (-35.2276, -41.0215) (-35.199, -41.0325) (-35.14, -41.0474) (-35.1044, -41.0474) knots 0 0 0 1 2 2 2
  spline S67 degree 2 poles (-35.1044, -41.0474) (-35.0733, -41.0474) (-35.0007, -41.0318) (-34.9786, -41.0111) knots 0 0 0 1 2 2 2
  spline S68 degree 2 poles (-34.9786, -41.0111) (-34.9624, -40.9949) (-34.9443, -40.9553) (-34.9443, -40.9223) knots 0 0 0 1 2 2 2
  spline S69 degree 2 poles (-34.9443, -40.9223) (-34.9443, -40.8938) (-34.9676, -40.8536) (-34.9864, -40.8412) knots 0 0 0 1 2 2 2
  spline S70 degree 2 poles (-34.9864, -40.8412) (-35.0136, -40.8231) (-35.0914, -40.8127) (-35.1193, -40.8127) knots 0 0 0 1 2 2 2
  spline S71 degree 2 poles (-35.1193, -40.8127) (-35.1634, -40.8127) (-35.247, -40.827) (-35.2775, -40.8348) knots 0 0 0 1 2 2 2
  line L335 (-35.2775, -40.8348) -> (-35.295, -40.8348)
  line L336 (-35.295, -40.8348) -> (-35.295, -40.3855)
  line L337 (-35.295, -40.3855) -> (-34.7647, -40.3855)
  line L338 (-34.7647, -40.3855) -> (-34.7647, -40.5365)
  line L339 (-34.7647, -40.5365) -> (-35.105, -40.5365)
  line L340 (-35.105, -40.5365) -> (-35.105, -40.6694)
  spline S72 degree 2 poles (-35.105, -40.6694) (-35.0888, -40.6681) (-35.0441, -40.6668) (-35.0318, -40.6668) knots 0 0 0 1 2 2 2
  spline S73 degree 2 poles (-35.0318, -40.6668) (-34.9741, -40.6668) (-34.8768, -40.6902) (-34.8386, -40.7142) knots 0 0 0 1 2 2 2
  spline S74 degree 2 poles (-34.8386, -40.7142) (-34.7932, -40.744) (-34.7426, -40.8432) (-34.7426, -40.9145) knots 0 0 0 1 2 2 2
  line L341 (34.3688, -41.2453) -> (34.1678, -41.2453)
  line L342 (34.1678, -41.2453) -> (34.1678, -40.8907)
  line L343 (34.1678, -40.8907) -> (33.8949, -40.8907)
  line L344 (33.8949, -40.8907) -> (33.8949, -41.2453)
  line L345 (33.8949, -41.2453) -> (33.6939, -41.2453)
  line L346 (33.6939, -41.2453) -> (33.6939, -40.4453)
  line L347 (33.6939, -40.4453) -> (33.8949, -40.4453)
  line L348 (33.8949, -40.4453) -> (33.8949, -40.7384)
  line L349 (33.8949, -40.7384) -> (34.1678, -40.7384)
  line L350 (34.1678, -40.7384) -> (34.1678, -40.4453)
  line L351 (34.1678, -40.4453) -> (34.3688, -40.4453)
  line L352 (34.3688, -40.4453) -> (34.3688, -41.2453)
  spline S75 degree 2 poles (35.1163, -40.9731) (35.1163, -41.0995) (34.9561, -41.2622) (34.8161, -41.2622) knots 0 0 0 1 2 2 2
  spline S76 degree 2 poles (34.8161, -41.2622) (34.7461, -41.2622) (34.6365, -41.222) (34.5983, -41.1825) knots 0 0 0 1 2 2 2
  spline S77 degree 2 poles (34.5983, -41.1825) (34.5529, -41.1364) (34.5043, -40.9906) (34.5043, -40.8888) knots 0 0 0 1 2 2 2
  spline S78 degree 2 poles (34.5043, -40.8888) (34.5043, -40.7838) (34.5497, -40.6204) (34.6009, -40.5575) knots 0 0 0 1 2 2 2
  spline S79 degree 2 poles (34.6009, -40.5575) (34.6495, -40.4979) (34.8077, -40.4304) (34.9159, -40.4304) knots 0 0 0 1 2 2 2
  spline S80 degree 2 poles (34.9159, -40.4304) (34.9555, -40.4304) (35.0346, -40.4408) (35.0488, -40.444) knots 0 0 0 1 2 2 2
  line L353 (35.0488, -40.444) -> (35.0488, -40.6009)
  line L354 (35.0488, -40.6009) -> (35.0346, -40.6009)
  spline S81 degree 2 poles (35.0346, -40.6009) (35.0203, -40.5938) (34.9555, -40.5763) (34.914, -40.5763) knots 0 0 0 1 2 2 2
  spline S82 degree 2 poles (34.914, -40.5763) (34.82, -40.5763) (34.7176, -40.6755) (34.7052, -40.7675) knots 0 0 0 1 2 2 2
  spline S83 degree 2 poles (34.7052, -40.7675) (34.7448, -40.7423) (34.8258, -40.7124) (34.877, -40.7124) knots 0 0 0 1 2 2 2
  spline S84 degree 2 poles (34.877, -40.7124) (34.9205, -40.7124) (34.9963, -40.7358) (35.0255, -40.7578) knots 0 0 0 1 2 2 2
  spline S85 degree 2 poles (35.0255, -40.7578) (35.067, -40.7896) (35.1163, -40.8927) (35.1163, -40.9731) knots 0 0 0 1 2 2 2
  spline S86 degree 2 poles (34.8822, -41.0936) (34.8978, -41.0742) (34.9146, -41.0288) (34.9146, -40.9828) knots 0 0 0 1 2 2 2
  spline S87 degree 2 poles (34.9146, -40.9828) (34.9146, -40.9439) (34.8952, -40.8933) (34.8777, -40.8784) knots 0 0 0 1 2 2 2
  spline S88 degree 2 poles (34.8777, -40.8784) (34.8595, -40.8628) (34.8148, -40.8518) (34.7895, -40.8518) knots 0 0 0 1 2 2 2
  spline S89 degree 2 poles (34.7895, -40.8518) (34.7681, -40.8518) (34.724, -40.8628) (34.7046, -40.8706) knots 0 0 0 1 2 2 2
  spline S90 degree 2 poles (34.7046, -40.8706) (34.7046, -40.8758) (34.7033, -40.9004) (34.7033, -40.9192) knots 0 0 0 1 2 2 2
  spline S91 degree 2 poles (34.7033, -40.9192) (34.7033, -40.9886) (34.7273, -41.0722) (34.7461, -41.0936) knots 0 0 0 1 2 2 2
  spline S92 degree 2 poles (34.7461, -41.0936) (34.7597, -41.1111) (34.796, -41.1261) (34.8155, -41.1261) knots 0 0 0 1 2 2 2
  spline S93 degree 2 poles (34.8155, -41.1261) (34.8317, -41.1261) (34.8693, -41.1098) (34.8822, -41.0936) knots 0 0 0 1 2 2 2
  point P0 (0, 0)
  point P1 (-22.175, 0.25)
  point P2 (-22.175, 0.5)
  point P3 (0, 0.25)
  point P4 (0, 0.5)
  point P5 (22.175, 0.25)
  point P6 (22.175, 0.5)
  point P7 (14, 0)
  point P8 (0, -0.25)
  point P9 (-14, 0)
  point P10 (22.175, -0.25)
  point P11 (0, -0.5)
  point P12 (-22.175, -0.5)
  point P13 (-22.175, -0.25)
  point P14 (22.175, -0.5)
  point P15 (32.5, -45)
  point P16 (-32.5, -45)
  dimension "d52" = 7
  dimension "d53" = 0.25
  dimension "d54" = 0.25
  dimension "d55" = 0.25
  dimension "d56" = 0.25
  dimension "d57" = 0.25
  dimension "d58" = 0.25
  dimension "d59" = 0.25
  dimension "d60" = 0.075
  dimension "d63" = 360
  dimension "d65" = 0.075
  dimension "d66" = 0.075
  constraints: 218 end point, 24 perpendicular, 18 centre point, 18 point on line, 15 equal radius, 7 parallel, 6 coincident, 6 midpoint, 4 equal length, 3 horizontal, 3 vertical alignment, 288 other
  measures "d52" diameter of A22
  measures "d53" distance between parallel lines of L21 L44
  measures "d54" distance between parallel lines of L41 L20
  measures "d55" distance between parallel lines of L19 L42
  measures "d56" distance between parallel lines of L14 L45
  measures "d57" distance between parallel lines of L61 L57
  measures "d58" distance between parallel lines of L62 L56
  measures "d59" distance between parallel lines of L63 L55
  measures "d60" distance between parallel lines of L55 L66
  measures "d65" radial gap between concentric circles of A22 A31
  measures "d66" radial gap between concentric circles of A32 A22
extrude "Extrusion4" add sketch "Sketch6" along normal blind 0.055 contours L87 L86 L85 L84 L101 L100 L99 L98 L97 L96 L18 L78 L79 L80 L81 L82 L83 L66 L67 L68 L69 L4 | L4 L70 L6 L88 | L6 L70 L71 L72 L73 L10 L91 L90 L89 L88 | L10 L74 L12 L92 | L12 L74 L75 L76 L77 L16 L95 L94 L93 L92 | L96 L16 L78 L18 | L130 L133 L136 L146 L140 L150 L137 L153 L106 L104 L38 L103 L105 L151 L142 L148 L138 L145 L134 L131 L141 L22 | L22 L141 L26 L130 | L26 L111 L154 L156 L122 L28 L117 L114 L155 L109 | L28 L122 L32 L117 | L32 L121 L120 L116 L115 L34 L127 L147 L119 L118 | L34 L115 L38 L127 | A31 | A33 | A35 | A37 | A39 | A41 | L189 L190 L191 L192 L193 L194 L195 L196 L197 L198 L199 L200 | L201 L202 L203 L204 L205 L206 S0 S1 L207 L208 L209 L210 | L211 L212 L213 L214 L215 L216 L217 L218 L219 L220 L221 L222 | L223 L224 S2 S3 S4 S5 S6 L225 L226 S7 S8 S9 S10 L227 L228 | L229 L230 L231 L232 L233 L234 L235 L236 L237 L238 L239 L240 | L241 L242 L243 L244 L245 L246 L247 L248 L249 L250 L251 | L255 L256 L257 L258 L259 L260 L261 L262 L263 L264 L265 L266 | S11 S12 S13 L267 L268 S14 S15 S16 S17 S18 L269 L270 L271 S19 S20 S21 S22 S23 S24 L272 L273 S25 S26 S27 S28 L274 S29 S30 | S31 S32 S33 L275 L276 L277 L278 L279 S34 S35 | L283 L284 L285 L286 L287 L288 L289 | L290 L291 S41 S42 S43 S44 S45 L292 L293 S46 S47 S48 S49 L294 L295 | S50 S51 S52 L296 L297 L298 L299 L300 S53 S54 | L304 L305 L306 L307 L308 L309 L310 | L311 L312 L313 L314 L315 L316 S60 S61 L317 L318 L319 L320 | L321 L322 L323 L324 L325 L326 L327 L328 L329 L330 L331 L332 | S62 S63 S64 L333 L334 S65 S66 S67 S68 S69 S70 S71 L335 L336 L337 L338 L339 L340 S72 S73 S74 | L341 L342 L343 L344 L345 L346 L347 L348 L349 L350 L351 L352 | S75 S76 S77 S78 S79 S80 L353 L354 S81 S82 S83 S84 S85
equation "\"d54\" = d53"
equation "\"d55\" = d53"
equation "\"d56\" = d53"
equation "\"d57\" = d53"
equation "\"d58\" = d53"
equation "\"d59\" = d53"
equation "\"d65\" = d60"
equation "\"d66\" = d65"
body "Solid1"
